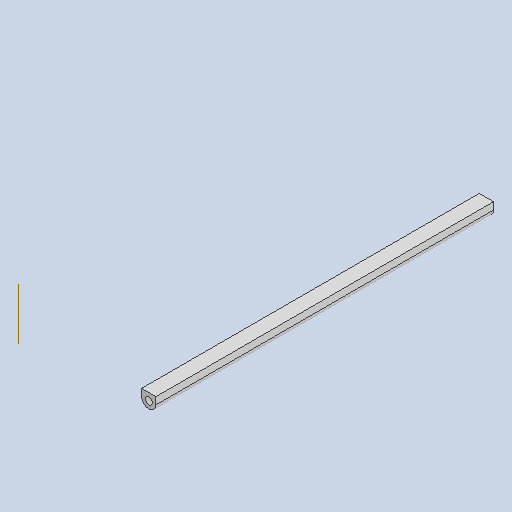
# Autodesk Inventor part: BaseShaft
Saved by Autodesk Inventor 2025.1 (Build 291241000, 241)
## iProperties
Created: 2026-05-10
Part Number: BaseShaft
Material: Generic
Document SubType Name: Modeling
Designer: User
Density: 1 g/cm^3
Appearance: Default
Author: User
## iProperties of the stored document BaseShaft_3DPrint.ipt
Created: 2026-05-11
Part Number: BaseShaft_3DPrint
Material: Generic
Document SubType Name: Modeling
Designer: User
Density: 1 g/cm^3
Appearance: Default
Author: User
Autodesk Inventor part; units mm, degrees
ref_plane "YZ Plane" through (0, 0, 0) normal (1, 0, 0) x (0, 1, 0)
ref_plane "XZ Plane" through (0, 0, 0) normal (0, 1, 0) x (-1, 0, 0)
ref_plane "Work Plane1" through (0, 0, 0) normal (0, 0, 1) x (1, 0, 0)
sketch "Sketch1" plane through (0, 0, 0) normal (0, 0, 1) x (1, 0, 0)
  line L0 (28.2, -13.1349) -> (28.2, -18.3349) projected
  arc A0 (17.8, -18.3349) -> (28.2, -18.3349) centre (23, -18.3349) ccw projected
  line L1 (17.8, -18.3349) -> (17.8, -13.1349) projected
  line L2 (17.8, -13.1349) -> (28.2, -13.1349) projected
  line L3 (205.8753, -18.3349) -> (205.8753, -13.1349) projected
  line L4 (205.8753, -13.1349) -> (216.2753, -13.1349) projected
  line L5 (216.2753, -13.1349) -> (216.2753, -18.3349) projected
  arc A1 (205.8753, -18.3349) -> (216.2753, -18.3349) centre (211.0753, -18.3349) ccw projected
  line L6 (226.007, -27.5) -> (182.0614, -27.5) projected
  line L7 (226.007, 5) -> (226.007, -27.5) projected
  line L8 (14, 5) -> (226.007, 5) projected
  line L9 (14, -27.5) -> (14, 5) projected
  line L10 (52.5458, -27.5) -> (14, -27.5) projected
  line L11 (105.8221, -25.5) -> (103.8221, -27.5) projected
  line L12 (105.8221, -25.5) -> (105.8221, -8.9699) projected
  line L13 (105.8221, -8.9699) -> (111.2221, -8.9699) projected
  line L14 (111.2221, -8.9699) -> (111.2221, -25.5) projected
  line L15 (113.2221, -27.5) -> (111.2221, -25.5) projected
  line L16 (151.8, -27.5) -> (113.2221, -27.5) projected
  line L17 (153.8, -25.5) -> (151.8, -27.5) projected
  line L18 (153.8, -25.5) -> (153.8, -8.9699) projected
  line L19 (153.8, -8.9699) -> (159.2, -8.9699) projected
  line L20 (159.2, -8.9699) -> (159.2, -19.6294) projected
  line L21 (216.0753, -18.3349) -> (216.0753, -13.3349)
  line L22 (216.0753, -13.3349) -> (206.0753, -13.3349)
  line L23 (206.0753, -13.3349) -> (206.0753, -18.3349)
  arc A2 (206.0753, -18.3349) -> (216.0753, -18.3349) centre (211.0753, -18.3349) ccw
  circle A3 centre (211.0753, -18.3349) radius 2.5
  line L24 (182.0614, -27.0054) -> (182.0614, -27.5) projected
  line L25 (52.5458, -27.5) -> (52.5458, -27.003) projected
  line L26 (52.5458, -27.003) -> (55.9407, -27.003) projected
  arc A4 (55.9407, -27.003) -> (66.5602, -14.9102) centre (55.9407, -16.2937) ccw projected
  line L27 (66.5602, -14.9102) -> (70.1135, -14.9102) projected
  line L28 (70.1135, -14.9102) -> (75.8231, -20.6198) projected
  arc A5 (72.9244, -27.5) -> (75.8231, -20.6198) centre (55.9407, -16.2937) ccw projected
  line L29 (103.8221, -27.5) -> (72.9244, -27.5) projected
  line L30 (159.2, -19.6294) -> (164.284, -14.5322) projected
  line L31 (164.284, -14.5322) -> (168.2242, -14.5271) projected
  arc A6 (168.2242, -14.5271) -> (178.6664, -27.0054) centre (178.6664, -16.397) ccw projected
  line L32 (178.6664, -27.0054) -> (182.0614, -27.0054) projected
  circle A7 centre (55.9407, -16.2937) radius 1.5 projected
  circle A8 centre (178.6664, -16.397) radius 1.5 projected
  point P0 (0, 0)
  dimension "d0" = 0.2
  dimension "d1" = 5
  constraints: 6 end point, 2 centre point, 2 point on circle, 1 coincident, 3 other
  measures "d0" radial gap between concentric circles of A1 A2
  measures "d1" diameter of A3
ref_plane "Work Plane2" through (14, -27.5, -235.8278) normal (0, 0, -1) x (0, 1, 0)
extrude "Extrusion1" add sketch "Sketch1" against normal up to surface (235.8278 mm away) contours A2 L23 L22 L21
body "Solid1"
